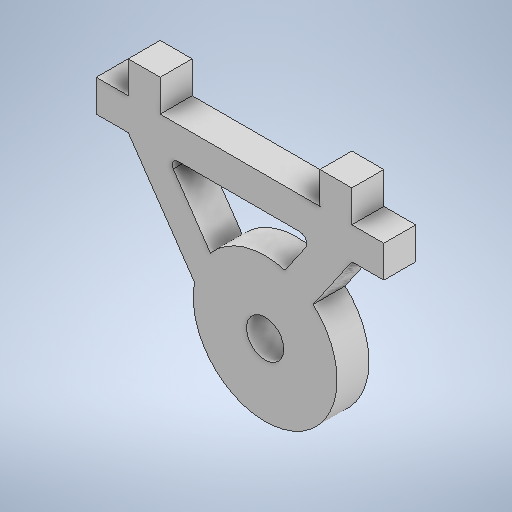
# Autodesk Inventor part: RODAl
Saved by Autodesk Inventor 2025.1 (Build 291241000, 241)
## iProperties
Created: 2024-10-25
Part Number: RODAl
Material: Genérico
Document SubType Name: Modeling
Designer: ambrosildo
Density: 1 g/cm^3
Appearance: Padrão
Author: ambrosildo
Autodesk Inventor part; units mm, degrees
ref_plane "YZ Plane" through (0, 0, 0) normal (1, 0, 0) x (0, 1, 0)
ref_plane "XZ Plane" through (0, 0, 0) normal (0, 1, 0) x (-1, 0, 0)
ref_plane "XY Plane" through (0, 0, 0) normal (0, 0, 1) x (1, 0, 0)
sketch "Esboço1" plane through (0, 0, 0) normal (0, 0, 1) x (1, 0, 0)
  line L0 (-13.5, 0) -> (0, 0)
  line L1 (-13.5, -3) -> (-13.5, 0)
  circle A0 centre (2.3584, -13.3187) radius 1.75
  arc A1 (-5.8288, -3) -> (-6.2756, -3.8492) centre (-5.8288, -3.5421) ccw
  line L2 (-13.5, -3) -> (-10.5, -3)
  line L3 (-6.2756, -3.8492) -> (-2.777, -8.938)
  line L4 (-10.5, -3) -> (-4.2728, -12.0577)
  line L5 (13.5, 0) -> (0, 0)
  line L6 (13.5, -3) -> (13.5, 0)
  line L7 (13.5, -3) -> (10.5, -3)
  line L8 (6.1478, -4.035) -> (4.225, -6.8319)
  arc A2 (6.1478, -4.035) -> (5.6034, -3) centre (5.6034, -3.6607) ccw
  line L9 (0, -3) -> (-5.8288, -3)
  line L10 (-10.5, -3) -> (-13.5, -3)
  line L11 (0, -3) -> (5.6034, -3)
  line L12 (10.5, -3) -> (13.5, -3)
  line L13 (10.5, -3) -> (6.8624, -8.2911)
  arc A3 (4.225, -6.8319) -> (-2.777, -8.938) centre (2.3584, -13.3187) ccw
  arc A4 (-4.2728, -12.0577) -> (6.8624, -8.2911) centre (2.3584, -13.3187) ccw
  point P0 (-6.8594, -3)
  point P1 (6.8594, -3)
  dimension "d0" = 3.5
  dimension "d1" = 3
  dimension "d2" = 3
  dimension "d3" = 3
  constraints: 28 end point, 8 point on circle, 7 tangent, 5 centre point, 3 parallel, 1 coincident, 1 horizontal
  measures "d0" diameter of A0
  measures "d1" distance of L1.start L4.start
  measures "d2" distance between parallel lines of L3 L4
  measures "d3" distance of L1.start L0.start
extrude "Extrusão1" add sketch "Esboço1" along normal blind 3
sketch "Esboço2" plane through (-13.5, 0, 0) normal (0, 1, 0) x (1, 0, 0)
  line L0 (0, 0) -> (3, 0) projected
  line L1 (3, 0) -> (6, 0)
  line L2 (6, 0) -> (6, -3)
  line L3 (6, -3) -> (3, -3)
  line L4 (3, -3) -> (3, 0)
  line L5 (27, 0) -> (0, 0) projected
  line L6 (24, 0) -> (21, 0)
  line L7 (21, 0) -> (21, -3)
  line L8 (21, -3) -> (24, -3)
  line L9 (24, -3) -> (24, 0)
  point P0 (13.5, 0)
  dimension "d6" = 3
  dimension "d7" = 3
  dimension "d9" = 3
  dimension "d10" = 3
  constraints: 16 end point, 4 parallel, 2 horizontal, 2 perpendicular, 1 point on line
  measures "d6" distance of L2.end L3.end
  measures "d7" distance of L1.end L2.end
  measures "d9" distance of L8.end L7.end
  measures "d10" distance of L7.end L6.end
extrude "Extrusão2" add sketch "Esboço2" along normal blind 3
